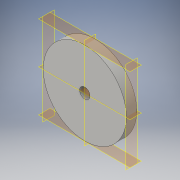
# Autodesk Inventor part: Intake Roller
Saved by Autodesk Inventor 2016 (Build 200138000, 138)
## iProperties
Created: 2016-01-16
Part Number: Intake Roller
Material: Generic
Document SubType Name: Modeling
Designer: Mentor1102
Density: 1 g/cm^3
Appearance: Default
Author: Mentor1102
Autodesk Inventor part; units mm, degrees
ref_plane "XY Plane" through (0, 0, 0) normal (0, 0, 1) x (1, 0, 0)
sketch "Sketch1" plane through (0, 0, 0) normal (0, 0, 1) x (1, 0, 0)
  circle A0 centre (0, 0) radius 6.35
  circle A1 centre (0, 0) radius 50.8
  dimension "d0" = 12.7
  dimension "d1" = 101.6
  constraints: 2 centre point, 2 coincident
  measures "d0" diameter of A0
  measures "d1" diameter of A1
extrude "Extrusion1" add sketch "Sketch1" along normal blind 12.7
ref_plane "Work Plane1" through (50.8, 0, 0) normal (1, 0, 0) x (0, 1, 0)
ref_plane "Work Plane2" through (-50.8, 0, 0) normal (1, 0, 0) x (0, 1, 0)
ref_plane "Work Plane3" through (0, 50.8, 0) normal (0, 1, 0) x (-1, 0, 0)
ref_plane "Work Plane4" through (0, -50.8, 0) normal (0, 1, 0) x (-1, 0, 0)
body "Solid1"
